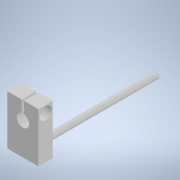
# Autodesk Inventor part: 4186566 DPDM 16-50---(p)
Saved by Autodesk Inventor 2021 (Build 250183000, 183)
## iProperties
Created: 2026-04-25
Part Number: 4186566 DPDM 16-50---(p)
Material: Generic
Catalog Web Link: www.3dfindit.com
Description: DPDM(p)-Guide plate
Vendor: FESTO
Document SubType Name: Modeling
Designer: psAdmin
Manufacturer: FESTO
Mass: 2.53206 g
Surface Area: 20.6682 cm^2
Volume: 2.53206 cm^3
Density: 1 g/cm^3
Appearance: PSOLRGB-176-176-176
Category: PARTsolutions
Company: FESTO
Title: 4186566 DPDM 16-50---(p)
Author: Cadenas PARTsolutions
Comments: Guide plate
PSOL_IDENT_0: {$CADENAS_DATA/23d-libs/festo/parts/d/dpdm/parts/dpdm_plate.prj},195 {VTYP=3D},{NB=4186566 DPDM 16-5
PSOL_IDENT_1: 0---(p)},{LINA=4186566 DPDM 16-50---(p)},{NN=DPDM(p)},{DATE=11.01.2023 08:49:49},{GEOMDATE=05.09.201
PSOL_IDENT_2: 9 13:41:48},{VERSION=},{LINEID=30},{WBVAR=HUB},{WBNUMERIC=HUB}  {NB=4186566 DPDM 16-50---(p)},{LINA=
PSOL_IDENT_3: 4186566 DPDM 16-50---(p)},{KT=DUMMY},{TNR=4186566},{TYP=DPDM},{KOL=16},{HUB=50},{HUB1=5,10,15,20,25,
PSOL_IDENT_4: 30,40,50},{B3=15.000},{H4=15.500},{H5=24.000},{MM=6.000},{H6=3.500},{LR=15.000},{DR=3.000},{Y1=13.30
PSOL_IDENT_5: 0}
NB: 4186566 DPDM 16-50---(p)
NN: DPDM(p)
NT: Guide plate
NBSYN: $TNR. $TYP. $KOL.-$HUB.---(p)
LINA: 4186566 DPDM 16-50---(p)
CATALOG: Festo
TNR: 4186566
TYP: DPDM
KOL: 16
HUB: 50
B3: 15
H4: 15.5
H5: 24
MM: 6
H6: 3.5
LR: 15
DR: 3
Y1: 13.3
SUPPLIER: FESTO
ARTICLENO: 4186566 DPDM 16-50---(p)
BOMINFO: 4186566 DPDM 16-50---(p)
CREATOR: CADENAS GmbH
Autodesk Inventor part; units mm, degrees
sketch "Sketch_1" plane through (0, 0, 0) normal (0, 0, 1) x (1, 0, 0)
  line L0 (-7.5, 24) -> (-7.5, 0)
  line L1 (-7.5, 0) -> (7.5, 0)
  line L2 (7.5, 0) -> (7.5, 24)
  line L3 (7.5, 24) -> (-7.5, 24)
  constraints: 8 end point
extrude "Extrusion1" add sketch "Sketch_1" against normal blind 7
sketch "Sketch_3" plane through (0, 0, 0) normal (0, 0, 1) x (1, 0, 0)
  arc A0 (-0.5, 18.458) -> (0.5, 18.458) centre (0, 15.5) ccw
  line L0 (0.5, 18.458) -> (0.5, 24)
  line L1 (0.5, 24) -> (-0.5, 24)
  line L2 (-0.5, 24) -> (-0.5, 18.458)
  constraints: 6 end point, 2 point on circle, 1 centre point
extrude "Extrusion2" cut sketch "Sketch_3" against normal blind 7
sketch "Sketch3" plane through (7.5, 0, 0) normal (1, 0, 0) x (0, 0, -1)
  point P0 (3.5, 20.5)
hole "Hole1" at (7.5, 20.5, -3.5) direction (-1, 0, 0) diameter 3.4 depth 7.5 counterbore diameter 5.9 counterbore depth 3.5
sketch "Sketch4" plane through (-7.5, 0, 0) normal (-1, 0, 0) x (0, 0, 1)
  point P0 (-3.5, 20.5)
hole "Hole2" at (-7.5, 20.5, -3.5) direction (1, 0, 0) diameter 2.459 depth 7 thread size "M3x0.5" class "6H" standard "ISO Metric profile"
sketch "Sketch_6" plane through (0, 0, 0) normal (1, 0, 0) x (0, 1, 0)
  line L0 (2.2, -65) -> (2.2, 0)
  line L1 (2.2, 0) -> (3.7, 0)
  line L2 (3.7, 0) -> (3.7, -64.6)
  line L3 (3.7, -64.6) -> (3.3, -65)
  line L4 (3.3, -65) -> (2.2, -65)
  line L5 (2.2, -65) -> (2.2, 0)
  constraints: 12 end point
revolve "Revolution1" add sketch "Sketch_6" angle 360 about axis through (0, 2.2, -65) along (0, 0, -1)
ref_plane "CP_PLATE_XY" through (0, 15.5, 0) normal (0, 0, 1) x (1, 0, 0)
ref_plane "CP_PLATE_YZ" through (0, 15.5, 0) normal (1, 0, 0) x (0, 1, 0)
ref_plane "CP_PLATE_ZX" through (0, 15.5, 0) normal (0, 1, 0) x (0, 0, 1)
ref_plane "CP_SCREW_XY" through (4, 20.5, -3.5) normal (1, 0, 0) x (0, 0, -1)
ref_plane "CP_SCREW_YZ" through (4, 20.5, -3.5) normal (0, 0, -1) x (0, 1, 0)
ref_plane "CP_SCREW_ZX" through (4, 20.5, -3.5) normal (0, 1, 0) x (1, 0, 0)
body "Solid1"
